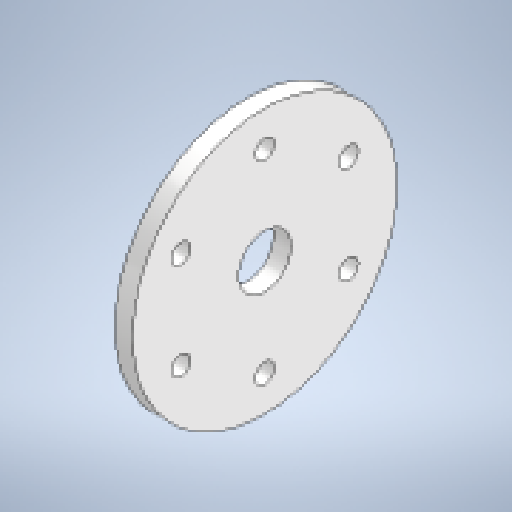
# Autodesk Inventor part: Wheel Cover
Saved by Autodesk Inventor 2023.2 (Build 272271000, 271)
## iProperties
Created: 2023-08-24
Part Number: Wheel Cover
Material: UHMW, White
Document SubType Name: Modeling
Designer: Nathan Cai
Mass: 5.14377 g
Surface Area: 41.3181 cm^2
Volume: 5.4721 cm^3
Density: 0.94 g/cm^3
Appearance: Smooth - White
Author: Nathan Cai
Autodesk Inventor part; units mm, degrees
ref_plane "YZ Plane" through (0, 0, 0) normal (1, 0, 0) x (0, 1, 0)
ref_plane "XZ Plane" through (0, 0, 0) normal (0, 1, 0) x (-1, 0, 0)
ref_plane "XY Plane" through (0, 0, 0) normal (0, 0, 1) x (1, 0, 0)
sketch "Sketch1" plane through (0, 0, 0) normal (1, 0, 0) x (0, 1, 0)
  circle A0 centre (0, 0) radius 23.8125
  circle A1 centre (0, 0) radius 17.4625 construction
  line L0 (0, 0) -> (23.8125, 0) construction
  circle A2 centre (17.4625, 0) radius 1.7526
  circle A3 centre (8.7313, 15.123) radius 1.7526
  circle A4 centre (-8.7312, 15.123) radius 1.7526
  circle A5 centre (-17.4625, 0) radius 1.7526
  circle A6 centre (-8.7313, -15.123) radius 1.7526
  circle A7 centre (8.7312, -15.123) radius 1.7526
  circle A8 centre (0, 0) radius 4.7625
  dimension "d0" = 47.625
  dimension "d1" = 34.925
  dimension "d2" = 3.5052
  dimension "d5" = 360
  dimension "d9" = 9.525
  constraints: 7 centre point, 3 coincident, 2 end point, 2 horizontal alignment, 1 horizontal, 1 point on line, 17 other
  measures "d2" diameter of A2
  measures "d9" diameter of A8
extrude "Extrusion1" add sketch "Sketch1" along normal blind 3.175
body "Solid1"
